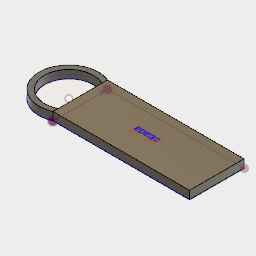
铭牌 (Autodesk Fusion 360 design; units mm, degrees)
Autodesk Fusion 360 part; units mm, degrees
sketch "草图3" plane through (0, 0, 0) normal (0, 1, 0) x (1, 0, 0)
  line L0 (0, 0) -> (-50, 0)
  line L1 (-50, 0) -> (-50, -20)
  line L2 (-50, -20) -> (0, -20)
  line L3 (0, -20) -> (0, 0)
extrude "拉伸2" add sketch "草图3" along normal blind 3 makes body 1
sketch "草图4" plane through (0, 0, 0) normal (0, 1, 0) x (1, 0, 0)
  arc A0 (-50, 0) -> (-50, -20) centre (-54.2, -10) ccw
  arc A1 (-50, -2.1375) -> (-50, -18) centre (-54.0808, -10.0688) ccw
  line L0 (-50, 0) -> (-50, -20)
  point P0 (-50, 0)
  point P1 (-50, -20)
extrude "拉伸3" add sketch "草图4" along normal blind 3 separate body contours A0 A1 L0 makes body 2
sketch "草图6" plane through (0, 0, 0) normal (0, 1, 0) x (1, 0, 0)
sketch "草图7" plane through (0, 0, 0) normal (0, 0, 1) x (1, 0, 0)
sketch "草图8" plane through (0, 3, 0) normal (0, 1, 0) x (-1, 0, 0)
  line L0 (0, 20) -> (0, 0)
  line L1 (0, 0) -> (50, 0)
  line L2 (50, 0) -> (50, 20)
  line L3 (50, 20) -> (0, 20)
  line L4 (21.3159, 8.9965) -> (29.7432, 8.9965) construction
  line L5 (29.7432, 8.9965) -> (29.7432, 11.9965) construction
  line L6 (29.7432, 11.9965) -> (21.3159, 11.9965) construction
  line L7 (21.3159, 11.9965) -> (21.3159, 8.9965) construction
sketch "草图5" plane through (0, 0, 0) normal (0, 1, 0) x (1, 0, 0)
  line L0 (-41.1284, -11.4325) -> (-11.6996, -16.6216) construction
  line L1 (-11.6996, -16.6216) -> (-9.9631, -6.7735) construction
  line L2 (-9.9631, -6.7735) -> (-39.3919, -1.5844) construction
  line L3 (-39.3919, -1.5844) -> (-41.1284, -11.4325) construction
extrude "拉伸4" [rolled back] along distance 6 taper angle 0
combine "合并1" [rolled back]
